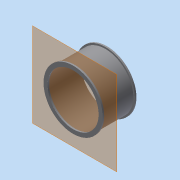
# Autodesk Inventor part: 01_Autofocus_10x_objective_copper_coil
Saved by Autodesk Inventor 2019.4 (Build 234330000, 330)
## iProperties
Created: 2020-11-23
Part Number: 01_Autofocus_10x_objective_copper_coil
Material: Generic
Document SubType Name: Modeling
Designer: diederichbenedict
Density: 1 g/cm^3
Appearance: Default
Author: diederichbenedict
Autodesk Inventor part; units mm, degrees
ref_plane "YZ Plane" through (0, 0, 0) normal (1, 0, 0) x (0, 1, 0)
ref_plane "XZ Plane" through (0, 0, 0) normal (0, 1, 0) x (-1, 0, 0)
ref_plane "XY Plane" through (0, 0, 0) normal (0, 0, 1) x (1, 0, 0)
ref_plane "Work Plane1" through (0, 0, -2) normal (0, 0, 1) x (-1, 0, 0)
sketch "Sketch1" plane through (0, 0, -2) normal (0, 0, 1) x (-1, 0, 0)
  circle A0 centre (0, 0) radius 8.1117 projected
  circle A1 centre (0, 0) radius 8.3117
  circle A2 centre (0, 0) radius 9.1117
  point P0 (0, 0)
  dimension "d0" = 0.2
  dimension "d1" = 1
  constraints: 2 centre point
  measures "d0" radial gap between concentric circles of A0 A1
  measures "d1" radial gap between concentric circles of A0 A2
extrude "Extrusion1" add sketch "Sketch1" against normal blind 10 contours A2
sketch "Sketch2" plane through (0, 0, -2) normal (0, 0, 1) x (1, 0, 0)
  circle A0 centre (0, 0) radius 8.3117 projected
  circle A1 centre (0, 0) radius 9.6318
  point P0 (0, 0)
  constraints: 1 centre point
extrude "Extrusion2" add sketch "Sketch2" along normal blind 0.5
sketch "Sketch3" plane through (0, 0, -12) normal (0, 0, -1) x (-1, 0, 0)
  circle A0 centre (0, 0) radius 9.6318 projected
  circle A1 centre (0, 0) radius 8.3117 projected
  point P0 (0, 0)
extrude "Extrusion3" add sketch "Sketch3" along normal blind 0.5
body "Solid1"
